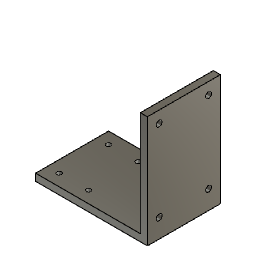
Camera Mount v1 (Autodesk Fusion 360 design; units mm, degrees)
Autodesk Fusion 360 part; units mm, degrees
sketch "Sketch1" plane through (0, 0, 0) normal (0, 0, 1) x (1, 0, 0)
  line L0 (-50, 25) -> (-2.5, 25)
  line L1 (-2.5, 25) -> (-2.5, -6)
  line L2 (-2.5, -6) -> (-50, -6)
  line L3 (-50, -6) -> (-50, 25)
  circle A0 centre (-45, 20) radius 1
  circle A1 centre (-32.5, 20) radius 1
  circle A2 centre (-45, -1) radius 1
  circle A3 centre (-32.5, -1) radius 1
  dimension "d1" = 2
  dimension "d2" = 2
  dimension "d3" = 2
  dimension "d4" = 2
  dimension "d5" = 12.5
  dimension "d6" = 5
  dimension "d7" = 5
  dimension "d8" = 12.5
  dimension "d9" = 21
  dimension "d10" = 21
  dimension "d11" = 5
  dimension "d12" = 5
  dimension "d13" = 5
  dimension "d14" = 5
  dimension "d15" = 30
  dimension "d16" = 47.5
  dimension "d17" = 31
  constraint horizontal L0
  constraint vertical L1
  constraint horizontal L2
  constraint vertical L3
  measures "d1" diameter of A0
  measures "d2" diameter of A1
  measures "d3" diameter of A2
  measures "d4" diameter of A3
  measures "d5" distance of A0.centre A1.centre
  measures "d6" distance of L0 A0.centre
  measures "d7" distance of L3 A0.centre
  measures "d8" distance of A2.centre A3.centre
  measures "d9" distance of A0.centre A2.centre
  measures "d10" distance of A1.centre A3.centre
  measures "d11" distance of L3 A2.centre
  measures "d12" distance of L2 A2.centre
  measures "d13" distance of L0 A1.centre
  measures "d14" distance of L2 A3.centre
  measures "d15" distance of L1 A1.centre
  measures "d16" distance of L0.start L0.end
  measures "d17" distance of L0.start L2.end
extrude "Extrude1" add sketch "Sketch1" along normal blind 3
sketch "Sketch2" plane through (0, 0, 3) normal (0, 0, 1) x (-1, 0, 0)
  circle A0 centre (45, 1) radius 1
  circle A1 centre (32.5, 1) radius 1
  circle A2 centre (32.5, -20) radius 1
  circle A3 centre (45, -20) radius 1
  line L0 (50, 6) -> (2.5, 6)
  line L1 (2.5, 6) -> (2.5, -25)
  line L2 (2.5, -25) -> (50, -25)
  line L3 (50, -25) -> (50, 6)
  line L4 (2.5, -25) -> (5.5, -25)
  line L5 (5.5, -25) -> (5.5, 6)
  line L6 (5.5, 6) -> (2.5, 6)
  line L7 (2.5, 6) -> (2.5, -25)
  dimension "d20" = 3
  dimension "d21" = 31
  constraint horizontal L4
  constraint vertical L5
  constraint horizontal L6
  constraint vertical L7
  constraint coincident L0 L5.end
  constraint coincident L1.end L2.start
  measures "d20" distance of L5 L7
  measures "d21" distance of L0.end L1.end
extrude "Extrude2" add sketch "Sketch2" along normal blind 44.5 contours L0 L1 L2 L4 L5 L6 L7
sketch "Sketch3" plane through (-5.5, 0, 0) normal (-1, 0, 0) x (0, -1, 0)
  line L0 (-25, 3) -> (6, 3)
  line L1 (6, 3) -> (6, 47.5)
  line L2 (6, 47.5) -> (-25, 47.5)
  line L3 (-25, 47.5) -> (-25, 3)
  circle A0 centre (-20, 42.5) radius 1.25
  circle A1 centre (1, 42.5) radius 1.25
  circle A2 centre (-20, 8) radius 1.25
  circle A3 centre (1, 8) radius 1.25
  dimension "d24" = 2.5
  dimension "d25" = 2.5
  dimension "d26" = 2.5
  dimension "d27" = 2.5
  dimension "d28" = 5
  dimension "d29" = 5
  dimension "d30" = 5
  dimension "d31" = 5
  dimension "d32" = 5
  dimension "d33" = 5
  dimension "d34" = 5
  dimension "d35" = 5
  measures "d24" diameter of A0
  measures "d25" diameter of A1
  measures "d26" diameter of A2
  measures "d27" diameter of A3
  measures "d28" distance of L1 A1.centre
  measures "d29" distance of L2 A1.centre
  measures "d30" distance of L2 A0.centre
  measures "d31" distance of L3 A0.centre
  measures "d32" distance of L3 A2.centre
  measures "d33" distance of L0 A2.centre
  measures "d34" distance of L0 A3.centre
  measures "d35" distance of L1 A3.centre
extrude "Extrude3" cut sketch "Sketch3" against normal blind 3 contours A0 | A1 | A2 | A3
